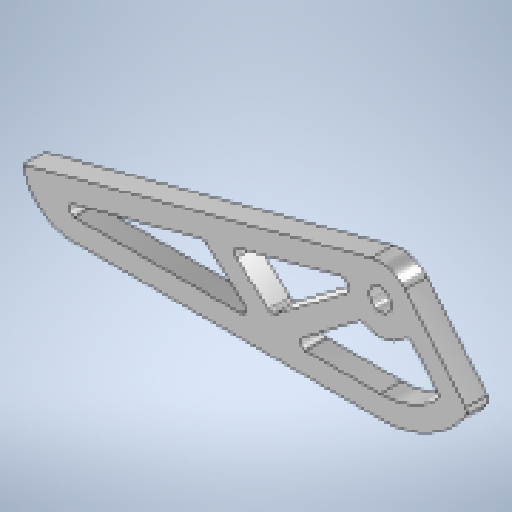
# Autodesk Inventor part: Arms
Saved by Autodesk Inventor 2023.2 (Build 272271000, 271)
## iProperties
Created: 2024-01-12
Part Number: Arms
Material: Aluminum 6061
Document SubType Name: Modeling
Designer: Nathan Cai
Mass: 36.3909 g
Surface Area: 80.0618 cm^2
Volume: 13.4781 cm^3
Density: 2.7 g/cm^3
Appearance: Aluminum - Flat
Author: Nathan Cai
Autodesk Inventor part; units mm, degrees
ref_plane "YZ Plane" through (0, 0, 0) normal (1, 0, 0) x (0, 1, 0)
ref_plane "XZ Plane" through (0, 0, 0) normal (0, 1, 0) x (-1, 0, 0)
ref_plane "XY Plane" through (0, 0, 0) normal (0, 0, 1) x (1, 0, 0)
sketch "Sketch1" plane through (0, 0, 0) normal (0, 0, 1) x (1, 0, 0)
  circle A0 centre (0, 0) radius 3.175
  arc A1 (0, -30.1625) -> (25.6926, -15.8009) centre (0, 0) ccw
  arc A2 (7.2966, 6.1226) -> (-2.4653, 9.2004) centre (0, 0) ccw
  line L0 (0, -30.1625) -> (-89.5849, -30.1625)
  circle A3 centre (0, 0) radius 105.5687 construction
  line L1 (7.2966, 6.1226) -> (25.6926, -15.8009)
  line L2 (0, 0) -> (0, -30.1625) construction
  line L3 (-2.4653, 9.2004) -> (-104.0209, -18.0113)
  arc A4 (-104.0209, -18.0113) -> (-89.5849, -30.1625) centre (-89.5849, -15.5117) ccw
  line L4 (-94.6631, -22.0779) -> (-0.8218, 3.0668)
  arc A5 (2.4322, 2.0409) -> (-0.8218, 3.0668) centre (0, 0) ccw
  line L5 (2.4322, 2.0409) -> (17.6019, -16.0377)
  arc A6 (0, -23.8125) -> (17.6019, -16.0377) centre (0, 0) ccw
  line L6 (0, -23.8125) -> (-89.5849, -23.8125)
  arc A7 (-94.6631, -22.0779) -> (-89.5849, -23.8125) centre (-89.5849, -15.5117) ccw
  circle A8 centre (0, 0) radius 9.525
  line L7 (0, 0) -> (-31.75, -23.8125) construction
  line L8 (-31.75, -23.8125) -> (-47.7424, -9.5055) construction
  line L9 (-51.4069, -10.4874) -> (-36.512, -23.8125)
  line L10 (-44.078, -8.5237) -> (-31.5729, -19.7109)
  line L11 (-31.5729, -19.7109) -> (-9.0892, -2.8482)
  line L12 (-26.4583, -23.8125) -> (-5.2792, -7.9282)
  point P0 (8.2046, -4.8384)
  point P1 (-9.496, 0.7426)
  dimension "d4" = 211.1375
  dimension "d0" = 6.35
  dimension "d2" = 19.05
  dimension "d10" = 40
  dimension "d12" = 15
  dimension "d13" = 30.1625
  dimension "d14" = 6.35
  dimension "d15" = 31.75
  dimension "d16" = 3.175
  dimension "d17" = 3.175
  dimension "d18" = 3.175
  dimension "d19" = 3.175
  constraints: 26 end point, 14 point on circle, 8 centre point, 5 coincident, 5 point on line, 4 tangent, 2 midpoint, 2 parallel, 1 concentric, 1 horizontal, 9 other
  measures "d0" diameter of A0
  measures "d2" diameter of A2
  measures "d10" angle of L2 L1
  measures "d12" angle of L0 L3
  measures "d13" radius of A1
  measures "d14" distance between parallel lines of L3 L4
  measures "d15" horizontal distance of L7.end L7.start
  measures "d16" distance between parallel lines of L8 L9
  measures "d17" distance between parallel lines of L8 L10
  measures "d18" distance between parallel lines of L7 L12
  measures "d19" distance between parallel lines of L11 L7
extrude "Extrusion1" add sketch "Sketch1" along normal blind 6.35 contours A0 L5 A8 L4 | A0 L4 A8 A2 L5 | A8 L1 A1 L0 A4 L3 L4 A7 L6 A6 L5 | L12 L6 L9 L4 L10 L11 A8
fillet "Fillet2" radius 1.5875 12 edges at (-94.6631, -22.0779, 3.175) (-51.4069, -10.4874, 3.175) (-36.512, -23.8125, 3.175) (-31.5729, -19.7109, 3.175) (-44.078, -8.5237, 3.175) (-9.496, 0.7426, 3.175) (-9.0892, -2.8482, 3.175) (-5.2792, -7.9282, 3.175) (-26.4583, -23.8125, 3.175) (8.2046, -4.8384, 3.175) (17.6019, -16.0377, 3.175) (25.6926, -15.8009, 3.175)
equation "\"d4\" = 3.5 * d1"
equation "\"d17\" = d16"
equation "\"d18\" = d17"
equation "\"d19\" = d16"
equation "\"d1\" = 60.325"
body "Solid1"
